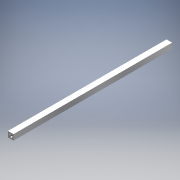
# Autodesk Inventor part: 2x2x1_8_tubeForLift
Saved by Autodesk Inventor 2018.2 (Build 222227000, 227)
## iProperties
Created: 2018-01-09
Part Number: 2x2x1_8_tubeForLift
Material: Aluminum 6061
Document SubType Name: Modeling
Designer: steele
Density: 2.7 g/cm^3
Appearance: Aluminum - Flat
Author: steele
Autodesk Inventor part; units mm, degrees
ref_plane "YZ Plane" through (0, 0, 0) normal (1, 0, 0) x (0, 1, 0)
ref_plane "XZ Plane" through (0, 0, 0) normal (0, 1, 0) x (-1, 0, 0)
ref_plane "XY Plane" through (0, 0, 0) normal (0, 0, 1) x (1, 0, 0)
sketch "Sketch1" plane through (0, 0, 0) normal (0, 0, 1) x (1, 0, 0)
  line L0 (-25.4, -25.4) -> (25.4, -25.4)
  line L1 (25.4, -25.4) -> (25.4, 25.4)
  line L2 (25.4, 25.4) -> (-25.4, 25.4)
  line L3 (-25.4, 25.4) -> (-25.4, -25.4)
  line L4 (-25.4, -25.4) -> (25.4, 25.4) construction
  line L5 (25.4, -25.4) -> (-25.4, 25.4) construction
  line L6 (-22.225, -22.225) -> (22.225, -22.225)
  line L7 (22.225, -22.225) -> (22.225, 22.225)
  line L8 (22.225, 22.225) -> (-22.225, 22.225)
  line L9 (-22.225, 22.225) -> (-22.225, -22.225)
  line L10 (-22.225, -22.225) -> (22.225, 22.225) construction
  line L11 (22.225, -22.225) -> (-22.225, 22.225) construction
  point P0 (0, 0)
  dimension "d0" = 50.8
  dimension "d1" = 50.8
  dimension "d2" = 3.175
  dimension "d3" = 3.175
  constraints: 24 end point, 5 parallel, 4 midpoint, 2 perpendicular, 1 horizontal
  measures "d0" distance of L0.start L0.end
  measures "d1" distance of L1.end L0.end
  measures "d2" distance between parallel lines of L6 L0
  measures "d3" distance between parallel lines of L3 L9
extrude "Extrusion1" add sketch "Sketch1" against normal blind 1447.8
sketch "Sketch2" plane through (0, 0, 0) normal (0, 0, 1) x (1, 0, 0)
  circle A0 centre (0, 0) radius 14.2875
  line L0 (-22.225, -22.225) -> (22.225, -22.225)
  line L1 (22.225, -22.225) -> (22.225, 22.225)
  line L2 (22.225, 22.225) -> (-22.225, 22.225)
  line L3 (-22.225, 22.225) -> (-22.225, -22.225)
  line L4 (-22.225, -22.225) -> (22.225, 22.225) construction
  line L5 (22.225, -22.225) -> (-22.225, 22.225) construction
  dimension "d6" = 28.575
  constraints: 12 end point, 2 midpoint, 2 parallel, 1 centre point, 1 coincident, 1 perpendicular
  measures "d6" diameter of A0
extrude "Extrusion2" add sketch "Sketch2" against normal blind 25.4
body "Solid1"
